Autodesk Fusion 360 part; units mm, degrees
note: some values were not read from the file. Set by a fixed rule: which sketch regions a step uses.
(part 2 of 2)
sketch "Skizze3" plane through (0, 0, -2) normal (0, 0, -1) x (1, 0, 0)
  circle A0 centre (-4.4364, 0.6745) radius 0.75
  circle A1 centre (-2, -0.5) radius 0.6
  circle A2 centre (0.5, -1) radius 0.6
  circle A3 centre (4.2471, 1.1495) radius 0.6
  circle A4 centre (6, -0.5) radius 0.6
  circle A5 centre (8.7313, 2.4606) radius 0.6
  circle A6 centre (6.5, 4) radius 0.6
  circle A7 centre (20.3684, 14.7264) radius 0.6
  circle A8 centre (15.5, 15.5) radius 0.6
  circle A9 centre (12.5896, 17.2675) radius 0.6
  circle A10 centre (9.5, 19.5) radius 0.6
  circle A11 centre (1.6733, 19.7308) radius 0.6
  circle A12 centre (2.9589, 23.7758) radius 0.6
  circle A13 centre (8.752, 22.7905) radius 0.6
  line L0 (16.328, 13.2614) -> (6.7681, 13.2342) construction
  line L1 (6.7681, 13.2342) -> (6.7821, 8.3103) construction
  line L2 (6.7821, 8.3103) -> (16.342, 8.3374) construction
  line L3 (16.342, 8.3374) -> (16.328, 13.2614) construction
  line L4 (6, 10) -> (10.7613, 12.7489) construction
  line L5 (6, 10) -> (8.7603, 8.4064) construction
  line L6 (6, 10) -> (17.8333, 10) construction
  arc A14 (3.1421, 11.65) -> (3.1421, 8.35) centre (6, 10) ccw
  arc A15 (0.9771, 12.9) -> (0.9771, 7.1) centre (6, 10) ccw
  arc A16 (-1.188, 14.15) -> (-1.188, 5.85) centre (6, 10) ccw
  arc A17 (5.3072, 10.4) -> (5.3072, 9.6) centre (6, 10) ccw
  arc A18 (4.2679, 11) -> (4.2679, 9) centre (6, 10) ccw
  arc A19 (2.1029, 12.25) -> (2.1029, 7.75) centre (6, 10) ccw
  arc A20 (-0.0622, 13.5) -> (-0.0622, 6.5) centre (6, 10) ccw
  arc A21 (-2.2272, 14.75) -> (-2.2272, 5.25) centre (6, 10) ccw
  line L7 (-1.188, 5.85) -> (-2.2272, 5.25) construction
  line L8 (-0.0622, 6.5) -> (0.9771, 7.1) construction
  line L9 (2.1029, 7.75) -> (3.1421, 8.35) construction
  line L10 (4.2679, 9) -> (5.3072, 9.6) construction
  line L11 (5.3072, 10.4) -> (4.2679, 11) construction
  line L12 (3.1421, 11.65) -> (2.1029, 12.25) construction
  line L13 (0.9771, 12.9) -> (-0.0622, 13.5) construction
  line L14 (-1.188, 14.15) -> (-2.2272, 14.75) construction
  arc A22 (4.2679, 9) -> (5.3072, 9.6) centre (4.7501, 9.3649) ccw
  arc A23 (2.1029, 7.75) -> (3.1421, 8.35) centre (2.6225, 8.05) ccw
  arc A24 (-0.066, 6.5067) -> (0.9771, 7.1) centre (0.4574, 6.8) ccw
  arc A25 (-2.2272, 5.25) -> (-1.188, 5.85) centre (-1.7076, 5.55) ccw
  arc A26 (5.3072, 10.4) -> (4.2679, 11) centre (4.7876, 10.7) ccw
  arc A27 (3.1421, 11.65) -> (2.1029, 12.25) centre (2.6225, 11.95) ccw
  arc A28 (0.9771, 12.9) -> (-0.0622, 13.5) centre (0.4574, 13.2) ccw
  arc A29 (-1.188, 14.15) -> (-2.2272, 14.75) centre (-1.7076, 14.45) ccw
  line L15 (7.7942, -9.2) -> (7.7942, 36.2) construction
  arc A30 (4.8827, -8) -> (8.1077, -8) centre (6.4952, -8.7) ccw
  line L16 (4.8827, -8) -> (8.1077, -8)
  line L17 (-4.6188, 23) -> (-8.9489, 23)
  line L18 (-8.9489, 23) -> (-11.4027, 18.75)
  line L19 (-11.4027, 18.75) -> (-9.2376, 15)
  line L20 (-9.2376, 15) -> (-11.4027, 11.25)
  line L21 (-11.4027, 11.25) -> (-9.2376, 7.5)
  line L22 (-9.2376, 7.5) -> (-11.4027, 3.75)
  line L23 (-11.4027, 3.75) -> (-8.9489, -0.5)
  line L24 (-8.9489, -0.5) -> (-4.6188, -0.5)
  line L25 (-4.6188, -0.5) -> (-2.4537, -4.25)
  line L26 (-2.4537, -4.25) -> (1.8764, -4.25)
  line L27 (1.8764, -4.25) -> (4.3444, -8.5248)
  arc A31 (4.3444, -8.5248) -> (8.6459, -8.5248) centre (6.4952, -8.7) ccw
  line L28 (8.6459, -8.5248) -> (11.114, -4.25)
  line L29 (11.114, -4.25) -> (15.4441, -4.25)
  line L30 (15.4441, -4.25) -> (17.6092, -0.5)
  line L31 (17.6092, -0.5) -> (21.9393, -0.5)
  line L32 (21.9393, -0.5) -> (24.393, 3.75)
  line L33 (24.393, 3.75) -> (22.228, 7.5)
  line L34 (22.228, 7.5) -> (24.393, 11.25)
  line L35 (24.393, 11.25) -> (22.228, 15)
  line L36 (22.228, 15) -> (24.393, 18.75)
  line L37 (24.393, 18.75) -> (21.9393, 23)
  line L38 (21.9393, 23) -> (17.6092, 23)
  line L39 (17.6092, 23) -> (15.4441, 26.75)
  line L40 (15.4441, 26.75) -> (11.114, 26.75)
  line L41 (11.114, 26.75) -> (8.9489, 30.5)
  line L42 (8.9489, 30.5) -> (4.0415, 30.5)
  line L43 (4.0415, 30.5) -> (1.8764, 26.75)
  line L44 (1.8764, 26.75) -> (-2.4537, 26.75)
  line L45 (-2.4537, 26.75) -> (-4.6188, 23)
  point P0 (6, 10)
  point P1 (4.7876, 10.7)
  point P2 (2.6225, 11.95)
  point P3 (0.4574, 13.2)
  point P4 (-1.7076, 14.45)
  point P5 (-1.7076, 5.55)
  point P6 (0.4574, 6.8)
  point P7 (2.6225, 8.05)
  point P8 (4.7876, 9.3)
  point P9 (5.3072, 9.6)
  point P10 (4.2679, 9)
  point P11 (3.1421, 8.35)
  point P12 (2.1029, 7.75)
  point P13 (0.9771, 7.1)
  point P14 (-0.0622, 6.5)
  point P15 (-1.188, 5.85)
  point P16 (-2.2272, 5.25)
  point P17 (6.4952, -8.7)
  dimension "d25" = 1.5
  dimension "d26" = 3.5
  dimension "d28" = 150
  dimension "d29" = 150
  dimension "d30" = 1.2
  dimension "d31" = 1.2
  dimension "d32" = 1.2
  dimension "d33" = 1.2
  dimension "d34" = 0.8
  dimension "d35" = 3.3
  dimension "d36" = 5.8
  dimension "d37" = 8.3
  dimension "d54" = 1.2
  text T0 "NFC" font "Arial" height 3.5 align left top in box 9.56 x 4.924 at (16.328, 13.2614) x (-0.999996, -0.002841) y (0.002841, -0.999996) spacing 1
  constraint equal A1 A2
  constraint equal A2 A3
  constraint equal A3 A6
  constraint equal A5 A6
  constraint equal A4 A5
  constraint equal A11 A12
  constraint equal A12 A13
  constraint equal A10 A13
  constraint equal A9 A10
  constraint equal A8 A9
  constraint equal A7 A8
  constraint coincident P0 L4.start
  constraint horizontal L6
  constraint coincident L4 P11
  constraint coincident L4 P13
  constraint coincident L4 P15
  constraint coincident L4 P9
  constraint coincident L4 P10
  constraint coincident L4 P12
  constraint coincident L4 P14
  constraint coincident L4 P16
  constraint coincident L5 A17.start
  constraint coincident L5 A18.start
  constraint coincident L5 A14.start
  constraint coincident L5 A19.start
  constraint coincident L5 A15.start
  constraint coincident L5 A20.start
  constraint coincident L5 A16.start
  constraint coincident L5 A21.start
  constraint coincident P9 A17.end
  constraint coincident P10 A18.end
  constraint coincident P11 A14.end
  constraint coincident P12 A19.end
  constraint coincident P13 A15.end
  constraint coincident P14 A20.end
  constraint coincident P15 A16.end
  constraint coincident P16 A21.end
  constraint midpoint P1 L11
  constraint midpoint P2 L12
  constraint midpoint P3 L13
  constraint midpoint P4 L14
  constraint midpoint P5 L7
  constraint midpoint P6 L8
  constraint midpoint P7 L9
  constraint midpoint P8 L10
  constraint coincident P7 A23.centre
  constraint coincident P6 A24.centre
  constraint coincident P1 A26.centre
  constraint coincident P2 A27.centre
  constraint coincident P3 A28.centre
  constraint coincident P4 A29.centre
  constraint coincident P5 A25.centre
  constraint equal A1 A11
  measures "d25" diameter of A0
  measures "d28" angle of L4 L6
  measures "d29" angle of L5 L6
  measures "d30" distance of A17 A18
  measures "d31" distance of A14 A19
  measures "d32" distance of A15 A20
  measures "d33" distance of A16 A21
  measures "d34" distance of P0 P9
  measures "d35" distance of P11 P0
  measures "d36" distance of P0 P13
  measures "d37" distance of P0 A16.end
  measures "d54" diameter of A1
extrude "Extrusion7" cut sketch "Skizze3" sketch "Skizze3" against normal blind 0.1 contours A0 | A1 | A2 | A3 | A4 | A5 | A6 | A7 | A8 | A9 | A10 | A11 | A12 | A13 | A14 A19 A23 A27 | A15 A20 A24 A28 | A16 A21 A25 A29 | A17 A18 A22 A26 of sketch 2 text T0
equation "d2 = d1 - 1.2 mm"
equation "d3 = ( d1 - d2 - 0 mm ) * 1.5 - ( d1 - d2 ) / 2"
equation "d29 = d28"
equation "d31 = d30"
equation "d32 = d30"
equation "d33 = d30"
equation "d35 = d34 + 2.5 mm"
equation "d36 = d35 + 2.5 mm"
equation "d37 = d36 + 2.5 mm"
equation "d45 = d1"
equation "d46 = d1 - 1.2 mm"
